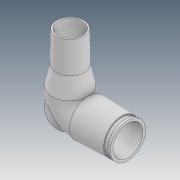
# Autodesk Inventor part: 90DegreeV3
Saved by Autodesk Inventor 2020 (Build 240168000, 168)
## iProperties
Created: 2020-04-13
Part Number: 90DegreeV3
Material: Generic
Document SubType Name: Modeling
Designer: Theo Cominotto
Density: 1 g/cm^3
Appearance: Default
Author: Theo Cominotto
Autodesk Inventor part; units mm, degrees
ref_plane "YZ Plane" through (0, 0, 0) normal (1, 0, 0) x (0, 1, 0)
sketch "Sketch1" plane through (0, 0, 0) normal (0, 0, 1) x (1, 0, 0)
  line L0 (0, 0) -> (0, 14.5) construction
  line L1 (0, 0) -> (31.6, 0) construction
  line L2 (31.6, 0) -> (31.6, 14) construction
  line L3 (0, 12.4997) -> (31.6, 11.9997)
  line L4 (0, 12.4997) -> (0, 14.5)
  line L5 (31.6, 14) -> (31.6, 11.9997)
  line L6 (29.6, 0) -> (29.6, 13.2) construction
  line L7 (29.6, 13.2) -> (29.6132, 14.0314)
  line L8 (29.6, 13.2) -> (26.4004, 13.2506)
  line L9 (26.4004, 13.2506) -> (26.4136, 14.0821)
  line L10 (31.6, 14) -> (29.6132, 14.0314)
  line L11 (26.4136, 14.0821) -> (0, 14.5)
  dimension "d0" = 14.5
  dimension "d1" = 31.6
  dimension "d2" = 14
  dimension "d4" = 13.2
  dimension "d5" = 2
  dimension "d6" = 3.2
  dimension "d22" = 2
  constraints: 24 end point, 5 perpendicular, 4 vertical, 3 point on line, 2 parallel, 1 collinear, 1 horizontal
  measures "d0" distance of L0.start L0.end
  measures "d1" distance of L0.start L1.end
  measures "d2" distance of L1.end L2.end
  measures "d4" distance of L6.start L6.end
  measures "d5" distance between parallel lines of L2 L6
  measures "d6" distance of L6.end L8.end
  measures "d22" distance between parallel lines of L10 L3
revolve "Revolution1" add sketch "Sketch1" angle 360 about axis through (0, 0, 0) along (1, 0, 0)
ref_plane "Work Plane1" through (0, 14.5, 0) normal (0, 1, 0) x (-1, 0, 0)
sketch "Sketch2" plane through (0, 14.5, 0) normal (0, 1, 0) x (-1, 0, 0)
  line L0 (0, 14.5) -> (0, -14.5) construction
  line L1 (0, 14.5) -> (0, -14.5) construction
  point P0 (0, 0)
  constraints: 2 end point, 1 collinear
sketch "Sketch3" plane through (0, 0, 0) normal (-1, 0, 0) x (0, 0, 1)
  circle A0 centre (0, 0) radius 14.5 projected
  circle A1 centre (0, 0) radius 12.4997 projected
revolve "Revolution2" add sketch "Sketch3" angle 90 about axis through (0, 14.5, 14.5) along (0, 0, -1)
sketch "Sketch4" plane through (0, 0, 0) normal (0, 0, 1) x (1, 0, 0)
  line L0 (0, 14.5) -> (-29, 14.5) construction
  line L1 (-14.5, 14.5) -> (0, 14.5) construction
  line L2 (0, 14.5) -> (26.4136, 14.0821) construction
  line L3 (-14.5, 14.5) -> (-14.5, 29.5) construction
  line L4 (-14.5, 29.5) -> (-3.25, 29.5) construction
  line L5 (-3.25, 29.5) -> (0, 14.5)
  line L6 (-14.5, 29.5) -> (-14.5, 54.5) construction
  line L7 (-14.5, 54.5) -> (-3.5, 54.5) construction
  line L8 (-3.5, 54.5) -> (-3.25, 29.5)
  line L9 (-3.5, 54.5) -> (-4.7, 54.5)
  line L10 (-4.7, 54.5) -> (-4.45, 29.5)
  line L11 (-4.45, 29.5) -> (-2.0003, 14.5)
  line L12 (-2.0003, 14.5) -> (0, 14.5)
  line L13 (-26.9997, 14.5) -> (-2.0003, 14.5) projected
  point P0 (0, 0)
  dimension "d10" = 15
  dimension "d11" = 11.25
  dimension "d12" = 25
  dimension "d13" = 11
  dimension "d14" = 1.2
  dimension "d15" = 1.2
  constraints: 22 end point, 4 point on line, 2 perpendicular, 2 vertical, 1 collinear, 1 horizontal, 1 midpoint
  measures "d10" distance of L1.start L3.end
  measures "d11" distance of L3.end L4.end
  measures "d12" distance of L3.end L6.end
  measures "d13" distance of L6.end L7.end
  measures "d14" distance of L7.end L9.end
  measures "d15" distance of L4.end L10.end
revolve "Revolution3" add sketch "Sketch4" angle 360 about axis through (-14.5, 29.5, 0) along (0, 1, 0)
ref_plane "Work Plane3" through (-19.799, -5.299, 14.5) normal (-0.7071068, -0.7071068, 0) x (0, 0, -1)
ref_plane "Work Plane2" through (0, 14.5, 14.5) normal (-0.7071068, -0.7071068, 0) x (0, 0, -1)
sketch "Sketch5" plane through (-19.799, -5.299, 14.5) normal (-0.7071068, -0.7071068, 0) x (0, 0, -1)
  circle A0 centre (14.5, 0) radius 14.5
  point P0 (14.5, 10.253)
  constraints: 1 centre point
extrude "Extrusion1" cut sketch "Sketch5" along normal blind 10
sketch "Sketch6" plane through (-19.799, -5.299, 14.5) normal (-0.7071068, -0.7071068, 0) x (-0.7071068, 0.7071068, 0)
  ellipse E0 centre (-10.253, 14.5) end of major axis (-10.253, 29) minor radius 10.253 projected
  circle A0 centre (0, 14.5) radius 12.5
  dimension "d23" = 25
  constraints: 1 centre point, 1 horizontal alignment, 1 other
  measures "d23" diameter of A0
extrude "Extrusion2" add sketch "Sketch6" against normal up to next contours A0 E0 | E0 A0 picked at (-4.1364, 16.63) picked at (3.9536, 16.6096)
sketch "Sketch7" plane through (0, 0, 0) normal (0, 0, 1) x (1, 0, 0)
  line L0 (0, 0) -> (0, 15) construction
  line L1 (0, -14.5) -> (0, 14.5) projected
  line L2 (0, 14.5) -> (0, 15)
  line L3 (31.6, -14) -> (31.6, 14) projected
  line L4 (0, 15) -> (31.6, 14)
  line L5 (26.4136, -14.0821) -> (26.4136, 14.0821) projected
  line L6 (26.4136, 14.0821) -> (26.4162, 14.164)
  line L7 (29.6132, -14.0314) -> (29.6132, 14.0314) projected
  line L8 (29.6132, 14.0314) -> (29.6141, 14.0628)
  line L9 (0, 14.5) -> (26.4136, 14.0821)
  line L10 (29.6132, 14.0314) -> (31.6, 14)
  line L11 (31.6, -11.9997) -> (31.6, 11.9997) projected
  line L12 (31.6, 0) -> (0, 0)
  dimension "d26" = 15
  constraints: 16 end point, 3 perpendicular, 2 collinear, 2 point on line, 1 midpoint, 1 vertical
  measures "d26" distance of L0.start L0.end
revolve "Revolution4" add sketch "Sketch7" angle 360 about axis through (31.6, 0, 0) along (-1, 0, 0) contours L2 L4 L6 L9 | L8 L4 L10
body "Solid1"
